Autodesk Inventor part; units mm, degrees
(part 2 of 3)
sketch "Эскиз30" plane through (0, 0, 0) normal (-1, 0, 0) x (0, 0, 1)
  circle A0 centre (-371.0468, 185.0848) radius 1.625 projected
  circle A1 centre (-103, 60) radius 2.1 projected
  circle A2 centre (-135.25, 60) radius 2.1 projected
  circle A3 centre (-173.9908, 56.343) radius 2.1 projected
  circle A4 centre (-50.8872, 165.0002) radius 2.1 projected
  circle A5 centre (-287, 56.343) radius 2.1 projected
  circle A6 centre (-319.1128, 165.0002) radius 2.1 projected
  arc A7 (-250, 372) -> (-253, 375) centre (-253, 372) ccw projected
  line L0 (-253, 375) -> (-377, 375) projected
  arc A8 (-377, 375) -> (-380, 372) centre (-377, 372) ccw projected
  line L1 (-380, 372) -> (-380, -2) projected
  arc A9 (-380, -2) -> (-377, -5) centre (-377, -2) ccw projected
  line L2 (-377, -5) -> (7, -5) projected
  arc A10 (7, -5) -> (10, -2) centre (7, -2) ccw projected
  line L3 (10, -2) -> (10, 372) projected
  arc A11 (10, 372) -> (7, 375) centre (7, 372) ccw projected
  line L4 (7, 375) -> (-117, 375) projected
  arc A12 (-117, 375) -> (-120, 372) centre (-117, 372) ccw projected
  line L5 (-120, 372) -> (-120, 323.5966) projected
  arc A13 (-123, 320.5966) -> (-120, 323.5966) centre (-123, 323.5966) ccw projected
  line L6 (-123, 320.5966) -> (-247, 320.5966) projected
  arc A14 (-250, 323.5966) -> (-247, 320.5966) centre (-247, 323.5966) ccw projected
  line L7 (-250, 323.5966) -> (-250, 372) projected
  arc A15 (-43, 338.848) -> (-40, 341.848) centre (-43, 341.848) ccw projected
  line L8 (-40, 341.848) -> (-40, 367) projected
  arc A16 (-37, 370) -> (-40, 367) centre (-37, 367) ccw projected
  line L9 (-37, 370) -> (-1, 370) projected
  arc A17 (2, 367) -> (-1, 370) centre (-1, 367) ccw projected
  line L10 (2, 367) -> (2, 269.848) projected
  arc A18 (-1, 266.848) -> (2, 269.848) centre (-1, 269.848) ccw projected
  line L11 (-1, 266.848) -> (-49, 266.848) projected
  arc A19 (-52, 269.848) -> (-49, 266.848) centre (-49, 269.848) ccw projected
  line L12 (-52, 269.848) -> (-52, 335.848) projected
  arc A20 (-49, 338.848) -> (-52, 335.848) centre (-49, 335.848) ccw projected
  line L13 (-49, 338.848) -> (-43, 338.848) projected
  arc A21 (-40, 28.152) -> (-43, 31.152) centre (-43, 28.152) ccw projected
  line L14 (-43, 31.152) -> (-49, 31.152) projected
  arc A22 (-52, 34.152) -> (-49, 31.152) centre (-49, 34.152) ccw projected
  line L15 (-52, 34.152) -> (-52, 100.152) projected
  arc A23 (-49, 103.152) -> (-52, 100.152) centre (-49, 100.152) ccw projected
  line L16 (-49, 103.152) -> (-43, 103.152) projected
  arc A24 (-43, 103.152) -> (-40, 106.152) centre (-43, 106.152) ccw projected
  line L17 (-40, 106.152) -> (-40, 160) projected
  arc A25 (-37, 163) -> (-40, 160) centre (-37, 160) ccw projected
  line L18 (-37, 163) -> (-1, 163) projected
  arc A26 (2, 160) -> (-1, 163) centre (-1, 160) ccw projected
  line L19 (2, 160) -> (2, 3) projected
  arc A27 (-1, 0) -> (2, 3) centre (-1, 3) ccw projected
  line L20 (-1, 0) -> (-37, 0) projected
  arc A28 (-40, 3) -> (-37, 0) centre (-37, 3) ccw projected
  line L21 (-40, 3) -> (-40, 28.152) projected
  line L22 (-165, 8) -> (-165, 44) projected
  arc A29 (-162, 47) -> (-165, 44) centre (-162, 44) ccw projected
  line L23 (-162, 47) -> (-96, 47) projected
  arc A30 (-93, 44) -> (-96, 47) centre (-96, 44) ccw projected
  line L24 (-93, 44) -> (-93, 8) projected
  arc A31 (-96, 5) -> (-93, 8) centre (-96, 8) ccw projected
  line L25 (-96, 5) -> (-162, 5) projected
  arc A32 (-165, 8) -> (-162, 5) centre (-162, 8) ccw projected
  circle A33 centre (-152.75, 251.9941) radius 2.1 projected
  circle A34 centre (-217.25, 118.0059) radius 2.1 projected
  circle A35 centre (-217.25, 57.0059) radius 2.1 projected
  circle A36 centre (-217.25, 251.9941) radius 2.1 projected
  circle A37 centre (-152.75, 312.9941) radius 2.1 projected
  circle A38 centre (-152.75, 118.0059) radius 2.1 projected
  circle A39 centre (-152.75, 57.0059) radius 2.1 projected
  circle A40 centre (-217.25, 312.9941) radius 2.1 projected
  circle A41 centre (-124.375, 193.0059) radius 2 projected
  circle A42 centre (-124.375, 129.0059) radius 2 projected
  line L26 (-98.825, 137.3849) -> (-98.825, 226.3849) projected
  arc A43 (-95.825, 229.3849) -> (-98.825, 226.3849) centre (-95.825, 226.3849) ccw projected
  line L27 (-95.825, 229.3849) -> (-87.825, 229.3849) projected
  arc A44 (-84.825, 226.3849) -> (-87.825, 229.3849) centre (-87.825, 226.3849) ccw projected
  line L28 (-84.825, 226.3849) -> (-84.825, 137.3849) projected
  arc A45 (-87.825, 134.3849) -> (-84.825, 137.3849) centre (-87.825, 137.3849) ccw projected
  line L29 (-87.825, 134.3849) -> (-95.825, 134.3849) projected
  arc A46 (-98.825, 137.3849) -> (-95.825, 134.3849) centre (-95.825, 137.3849) ccw projected
  line L30 (-358.5, 185.5001) -> (-358.5, 244.5001) projected
  arc A47 (-355.5, 247.5001) -> (-358.5, 244.5001) centre (-355.5, 244.5001) ccw projected
  line L31 (-355.5, 247.5001) -> (-335, 247.5001) projected
  arc A48 (-332, 244.5001) -> (-335, 247.5001) centre (-335, 244.5001) ccw projected
  line L32 (-332, 244.5001) -> (-332, 185.5001) projected
  arc A49 (-335, 182.5001) -> (-332, 185.5001) centre (-335, 185.5001) ccw projected
  line L33 (-335, 182.5001) -> (-355.5, 182.5001) projected
  arc A50 (-358.5, 185.5001) -> (-355.5, 182.5001) centre (-355.5, 185.5001) ccw projected
  line L34 (-35, 247.5001) -> (-14.5, 247.5001) projected
  arc A51 (-11.5, 244.5001) -> (-14.5, 247.5001) centre (-14.5, 244.5001) ccw projected
  line L35 (-11.5, 244.5001) -> (-11.5, 185.5001) projected
  arc A52 (-14.5, 182.5001) -> (-11.5, 185.5001) centre (-14.5, 185.5001) ccw projected
  line L36 (-14.5, 182.5001) -> (-35, 182.5001) projected
  arc A53 (-38, 185.5001) -> (-35, 182.5001) centre (-35, 185.5001) ccw projected
  line L37 (-38, 185.5001) -> (-38, 244.5001) projected
  arc A54 (-35, 247.5001) -> (-38, 244.5001) centre (-35, 244.5001) ccw projected
  arc A55 (-185, 192.7028) -> (-185, 193.309) centre (-183.175, 193.0059) ccw projected
  line L38 (-185, 192.7028) -> (-185, 193.309) projected
  circle A56 centre (-376, 368.9) radius 2.1 projected
  circle A57 centre (-299, 142) radius 1.625 projected
  circle A58 centre (-299, 2.0002) radius 1.625 projected
  circle A59 centre (-54, 368) radius 1.625 projected
  circle A60 centre (6, 1.1) radius 2.1 projected
  circle A61 centre (6, 368.9) radius 2.1 projected
  circle A62 centre (-54, 142) radius 1.625 projected
  circle A63 centre (1, 228) radius 1.625 projected
  circle A64 centre (-316, 2.0002) radius 1.625 projected
  circle A65 centre (-371, 228) radius 1.625 projected
  circle A66 centre (-299, 368) radius 1.625 projected
  circle A67 centre (-183.175, 129.0059) radius 1.85 projected
  circle A68 centre (-316, 228) radius 1.625 projected
  circle A69 centre (-316, 142) radius 1.625 projected
  circle A70 centre (-71, 228) radius 1.625 projected
  circle A71 centre (-71, 368) radius 1.625 projected
  circle A72 centre (-54, 2.0002) radius 1.625 projected
  circle A73 centre (-71, 2.0002) radius 1.625 projected
  circle A74 centre (-71, 142) radius 1.625 projected
  circle A75 centre (-54, 228) radius 1.625 projected
  circle A76 centre (-376, 1.1) radius 2.1 projected
  circle A77 centre (-299, 228) radius 1.625 projected
  circle A78 centre (-316, 368) radius 1.625 projected
  arc A79 (-330, 341.848) -> (-327, 338.848) centre (-327, 341.848) ccw projected
  line L39 (-327, 338.848) -> (-321, 338.848) projected
  arc A80 (-318, 335.848) -> (-321, 338.848) centre (-321, 335.848) ccw projected
  line L40 (-318, 335.848) -> (-318, 269.848) projected
  arc A81 (-321, 266.848) -> (-318, 269.848) centre (-321, 269.848) ccw projected
  line L41 (-321, 266.848) -> (-369, 266.848) projected
  arc A82 (-372, 269.848) -> (-369, 266.848) centre (-369, 269.848) ccw projected
  line L42 (-372, 269.848) -> (-372, 367) projected
  arc A83 (-369, 370) -> (-372, 367) centre (-369, 367) ccw projected
  line L43 (-369, 370) -> (-333, 370) projected
  arc A84 (-330, 367) -> (-333, 370) centre (-333, 367) ccw projected
  line L44 (-330, 367) -> (-330, 341.848) projected
  arc A85 (-327, 31.152) -> (-330, 28.152) centre (-327, 28.152) ccw projected
  line L45 (-330, 28.152) -> (-330, 3) projected
  arc A86 (-333, 0) -> (-330, 3) centre (-333, 3) ccw projected
  line L46 (-333, 0) -> (-369, 0) projected
  arc A87 (-372, 3) -> (-369, 0) centre (-369, 3) ccw projected
  line L47 (-372, 3) -> (-372, 160) projected
  arc A88 (-369, 163) -> (-372, 160) centre (-369, 160) ccw projected
  line L48 (-369, 163) -> (-333, 163) projected
  arc A89 (-330, 160) -> (-333, 163) centre (-333, 160) ccw projected
  line L49 (-330, 160) -> (-330, 106.152) projected
  arc A90 (-330, 106.152) -> (-327, 103.152) centre (-327, 106.152) ccw projected
  line L50 (-327, 103.152) -> (-321, 103.152) projected
  arc A91 (-318, 100.152) -> (-321, 103.152) centre (-321, 100.152) ccw projected
  line L51 (-318, 100.152) -> (-318, 34.152) projected
  arc A92 (-321, 31.152) -> (-318, 34.152) centre (-321, 34.152) ccw projected
  line L52 (-321, 31.152) -> (-327, 31.152) projected
  line L53 (-224.75, 65.0059) -> (-224.75, 110.0059) projected
  line L54 (-282, 51.343) -> (-282, 61.343) projected
  line L55 (-268.3252, 69.343) -> (-228.25, 69.343)
  line L56 (-226.25, 71.343) -> (-226.25, 99.9959)
  line L57 (-235.9248, 106.343) -> (-276, 106.343)
  line L58 (-278, 104.343) -> (-278, 75.6902)
  line L59 (-278, 69.343) -> (-226.25, 106.343)
  line L60 (-269.4885, 72.97) -> (-229.4132, 101.6228)
  line L61 (-274.8368, 74.0633) -> (-234.7615, 102.7161)
  arc A93 (-269.4885, 72.97) -> (-268.3252, 69.343) centre (-268.3252, 71.343) ccw
  arc A94 (-278, 75.6902) -> (-274.8368, 74.0633) centre (-276, 75.6902) ccw
  arc A95 (-234.7615, 102.7161) -> (-235.9248, 106.343) centre (-235.9248, 104.343) ccw
  arc A96 (-276, 106.343) -> (-278, 104.343) centre (-276, 104.343) ccw
  arc A97 (-228.25, 69.343) -> (-226.25, 71.343) centre (-228.25, 71.343) ccw
  arc A98 (-226.25, 99.9959) -> (-229.4132, 101.6228) centre (-228.25, 99.9959) ccw
  line L62 (-185, -235.3635) -> (-185, 601.2713)
  line L63 (-101.6748, 69.343) -> (-141.75, 69.343)
  line L64 (-143.75, 71.343) -> (-143.75, 99.9959)
  line L65 (-134.0752, 106.343) -> (-94, 106.343)
  line L66 (-92, 104.343) -> (-92, 75.6902)
  line L67 (-92, 69.343) -> (-143.75, 106.343)
  line L68 (-100.5115, 72.97) -> (-140.5868, 101.6228)
  line L69 (-95.1632, 74.0633) -> (-135.2385, 102.7161)
  arc A99 (-101.6748, 69.343) -> (-100.5115, 72.97) centre (-101.6748, 71.343) ccw
  arc A100 (-95.1632, 74.0633) -> (-92, 75.6902) centre (-94, 75.6902) ccw
  arc A101 (-134.0752, 106.343) -> (-135.2385, 102.7161) centre (-134.0752, 104.343) ccw
  arc A102 (-92, 104.343) -> (-94, 106.343) centre (-94, 104.343) ccw
  arc A103 (-143.75, 71.343) -> (-141.75, 69.343) centre (-141.75, 71.343) ccw
  arc A104 (-140.5868, 101.6228) -> (-143.75, 99.9959) centre (-141.75, 99.9959) ccw
  line L70 (-268.3252, 133.343) -> (-228.25, 133.343)
  line L71 (-226.25, 135.343) -> (-226.25, 163.9959)
  line L72 (-235.9248, 170.343) -> (-276, 170.343)
  line L73 (-278, 168.343) -> (-278, 139.6902)
  line L74 (-278, 133.343) -> (-226.25, 170.343)
  line L75 (-269.4885, 136.97) -> (-229.4132, 165.6228)
  line L76 (-274.8368, 138.0633) -> (-234.7615, 166.7161)
  arc A105 (-269.4885, 136.97) -> (-268.3252, 133.343) centre (-268.3252, 135.343) ccw
  arc A106 (-278, 139.6902) -> (-274.8368, 138.0633) centre (-276, 139.6902) ccw
  arc A107 (-234.7615, 166.7161) -> (-235.9248, 170.343) centre (-235.9248, 168.343) ccw
  arc A108 (-276, 170.343) -> (-278, 168.343) centre (-276, 168.343) ccw
  arc A109 (-228.25, 133.343) -> (-226.25, 135.343) centre (-228.25, 135.343) ccw
  arc A110 (-226.25, 163.9959) -> (-229.4132, 165.6228) centre (-228.25, 163.9959) ccw
  line L77 (-458.8698, 185) -> (88.8698, 185) projected
  line L78 (-268.3252, 300.657) -> (-228.25, 300.657)
  line L79 (-226.25, 298.657) -> (-226.25, 270.0041)
  line L80 (-235.9248, 263.657) -> (-276, 263.657)
  line L81 (-278, 265.657) -> (-278, 294.3098)
  line L82 (-278, 300.657) -> (-226.25, 263.657)
  line L83 (-269.4885, 297.03) -> (-229.4132, 268.3772)
  line L84 (-274.8368, 295.9367) -> (-234.7615, 267.2839)
  arc A111 (-268.3252, 300.657) -> (-269.4885, 297.03) centre (-268.3252, 298.657) ccw
  arc A112 (-274.8368, 295.9367) -> (-278, 294.3098) centre (-276, 294.3098) ccw
  arc A113 (-235.9248, 263.657) -> (-234.7615, 267.2839) centre (-235.9248, 265.657) ccw
  arc A114 (-278, 265.657) -> (-276, 263.657) centre (-276, 265.657) ccw
  arc A115 (-226.25, 298.657) -> (-228.25, 300.657) centre (-228.25, 298.657) ccw
  arc A116 (-229.4132, 268.3772) -> (-226.25, 270.0041) centre (-228.25, 270.0041) ccw
  line L85 (-134.0752, 263.657) -> (-94, 263.657)
  arc A117 (-94, 263.657) -> (-92, 265.657) centre (-94, 265.657) ccw
  arc A118 (-135.2385, 267.2839) -> (-134.0752, 263.657) centre (-134.0752, 265.657) ccw
  arc A119 (-143.75, 270.0041) -> (-140.5868, 268.3772) centre (-141.75, 270.0041) ccw
  line L86 (-92, 265.657) -> (-92, 294.3098)
  line L87 (-95.1632, 295.9367) -> (-135.2385, 267.2839)
  line L88 (-92, 300.657) -> (-143.75, 263.657)
  arc A120 (-100.5115, 297.03) -> (-101.6748, 300.657) centre (-101.6748, 298.657) ccw
  arc A121 (-92, 294.3098) -> (-95.1632, 295.9367) centre (-94, 294.3098) ccw
  line L89 (-101.6748, 300.657) -> (-141.75, 300.657)
  line L90 (-143.75, 298.657) -> (-143.75, 270.0041)
  arc A122 (-141.75, 300.657) -> (-143.75, 298.657) centre (-141.75, 298.657) ccw
  line L91 (-100.5115, 297.03) -> (-140.5868, 268.3772)
  arc A123 (-226.25, 230.3098) -> (-229.4132, 231.9367) centre (-228.25, 230.3098) ccw
  line L92 (-226.25, 201.657) -> (-226.25, 230.3098)
  arc A124 (-228.25, 199.657) -> (-226.25, 201.657) centre (-228.25, 201.657) ccw
  arc A125 (-278, 206.0041) -> (-274.8368, 204.3772) centre (-276, 206.0041) ccw
  arc A126 (-269.4885, 203.2839) -> (-268.3252, 199.657) centre (-268.3252, 201.657) ccw
  line L93 (-278, 234.657) -> (-278, 206.0041)
  arc A127 (-276, 236.657) -> (-278, 234.657) centre (-276, 234.657) ccw
  line L94 (-268.3252, 199.657) -> (-228.25, 199.657)
  line L95 (-235.9248, 236.657) -> (-276, 236.657)
  arc A128 (-234.7615, 233.03) -> (-235.9248, 236.657) centre (-235.9248, 234.657) ccw
  line L96 (-269.4885, 203.2839) -> (-229.4132, 231.9367)
  line L97 (-278, 199.657) -> (-226.25, 236.657)
  line L98 (-274.8368, 204.3772) -> (-234.7615, 233.03)
  arc A129 (-130.725, 234.2716) -> (-133.9769, 235.8314) centre (-132.725, 234.2716) ccw
  line L99 (-130.725, 206.0059) -> (-130.725, 234.2716)
  arc A130 (-138.3555, 237.4461) -> (-139.6074, 241.0059) centre (-139.6074, 239.0059) ccw
  line L100 (-167.9426, 204.0059) -> (-132.725, 204.0059)
  arc A131 (-169.1945, 207.5656) -> (-167.9426, 204.0059) centre (-167.9426, 206.0059) ccw
  line L101 (-169.1945, 207.5656) -> (-133.9769, 235.8314)
  line L102 (-176.825, 204.0059) -> (-130.725, 241.0059)
  line L103 (-173.5731, 209.1803) -> (-138.3555, 237.4461)
  line L104 (-139.6074, 241.0059) -> (-174.825, 241.0059)
  arc A132 (-176.825, 210.7401) -> (-173.5731, 209.1803) centre (-174.825, 210.7401) ccw
  line L105 (-176.825, 239.0059) -> (-176.825, 210.7401)
  arc A133 (-174.825, 241.0059) -> (-176.825, 239.0059) centre (-174.825, 239.0059) ccw
  arc A134 (-132.725, 204.0059) -> (-130.725, 206.0059) centre (-132.725, 206.0059) ccw
  line L106 (-130.725, 182.9338) -> (-130.725, 189.1279) projected
  point P0 (0, 0)
  point P1 (-145.25, 110.0059)
  point P2 (-255.9624, 106.343)
  point P3 (-224.75, 259.9941)
  point P4 (-145.25, 259.9941)
  point P5 (-255.9624, 263.657)
  point P6 (-226.25, 149.6695)
  point P7 (-176.825, 195.5059)
  dimension "d123" = 9
  dimension "d124" = 9
  dimension "d125" = 37
  dimension "d126" = 2
  dimension "d127" = 2
  dimension "d128" = 2
  dimension "d129" = 37
  dimension "d130" = 2
  dimension "d131" = 2
  dimension "d132" = 2
  dimension "d133" = 0
  dimension "d141" = 27
  dimension "d142" = 37
  dimension "d143" = 2
  dimension "d144" = 2
  dimension "d145" = 2
  dimension "d146" = 27
  dimension "d147" = 0
  dimension "d148" = 0
  dimension "d149" = 37
  dimension "d150" = 2
  dimension "d151" = 2
  dimension "d152" = 2
  dimension "d153" = 11
  dimension "d154" = 0
  dimension "d155" = 0
  constraints: 100 end point, 84 point on circle, 64 symmetric about line, 48 tangent, 42 centre point, 28 point on line, 20 equal radius, 16 parallel, 5 horizontal, 4 perpendicular, 2 midpoint, 1 vertical, 21 other
  measures "d123" distance from line of L58 A5.centre
  measures "d124" distance from line of A35.centre L56
  measures "d125" distance between parallel lines of L57 L55
  measures "d126" distance between parallel lines of L59 L60
  measures "d127" distance between parallel lines of L59 L61
  measures "d128" radius of A93
  measures "d129" distance between parallel lines of L72 L70
  measures "d130" distance between parallel lines of L74 L75
  measures "d131" distance between parallel lines of L74 L76
  measures "d132" radius of A105
  measures "d133" distance between parallel lines of L58 L73
  measures "d141" distance between parallel lines of L57 L70
  measures "d142" distance between parallel lines of L95 L94
  measures "d143" distance between parallel lines of L97 L96
  measures "d144" distance between parallel lines of L97 L98
  measures "d145" radius of A126
  measures "d146" distance between parallel lines of L95 L80
  measures "d147" distance between parallel lines of L73 L93
  measures "d148" distance from line of point (-226.25, 149.669) L92
  measures "d149" distance between parallel lines of L104 L100
  measures "d150" distance between parallel lines of L102 L101
  measures "d151" distance between parallel lines of L102 L103
  measures "d152" radius of A131
  measures "d153" distance from line of A55.centre L100
  measures "d154" distance from line of point (-176.825, 195.506) L105
  measures "d155" distance between parallel lines of L106 L99
extrude "Выдавливание27" cut sketch "Эскиз30" against normal blind 10 contours A93 L60 A98 L56 A97 L55 | A95 L61 A94 L58 A96 L57 | L63 A103 L64 A104 L68 A99 | L65 A102 L66 A100 L69 A101 | A105 L75 A110 L71 A109 L70 | A107 L76 A106 L73 A108 L72 | L78 A115 L79 A116 L83 A111 | L80 A114 L81 A112 L84 A113 | A118 L87 A121 L86 A117 L85 | L90 A122 L89 A120 L91 A119 | L92 A124 L94 A126 L96 A123 | L93 A127 L95 A128 L98 A125 | L99 A134 L100 A131 L101 A129 | L103 A132 L105 A133 L104 A130
sketch "Эскиз31" plane through (1.5, 0, 0) normal (1, 0, 0) x (0, 0, -1)
  point P0 (0, 0)
sketch "Эскиз32" plane through (1.5, 0, 0) normal (1, 0, 0) x (0, 0, -1)
  arc A0 (278, 234.657) -> (276, 236.657) centre (276, 234.657) ccw projected
  line L0 (278, 234.657) -> (278, 206.0041) projected
  arc A1 (274.8368, 204.3772) -> (278, 206.0041) centre (276, 206.0041) ccw projected
  line L1 (274.8368, 204.3772) -> (234.7615, 233.03) projected
  arc A2 (235.9248, 236.657) -> (234.7615, 233.03) centre (235.9248, 234.657) ccw projected
  line L2 (235.9248, 236.657) -> (276, 236.657) projected
  line L3 (278, 104.343) -> (278, 75.6902) projected
  arc A3 (274.8368, 74.0633) -> (278, 75.6902) centre (276, 75.6902) ccw projected
  line L4 (274.8368, 74.0633) -> (234.7615, 102.7161) projected
  arc A4 (235.9248, 106.343) -> (234.7615, 102.7161) centre (235.9248, 104.343) ccw projected
  line L5 (235.9248, 106.343) -> (276, 106.343) projected
  arc A5 (278, 104.343) -> (276, 106.343) centre (276, 104.343) ccw projected
  line L6 (176.825, 239.0059) -> (176.825, 210.7401) projected
  arc A6 (173.5731, 209.1803) -> (176.825, 210.7401) centre (174.825, 210.7401) ccw projected
  line L7 (173.5731, 209.1803) -> (138.3555, 237.4461) projected
  arc A7 (139.6074, 241.0059) -> (138.3555, 237.4461) centre (139.6074, 239.0059) ccw projected
  line L8 (139.6074, 241.0059) -> (174.825, 241.0059) projected
  arc A8 (176.825, 239.0059) -> (174.825, 241.0059) centre (174.825, 239.0059) ccw projected
  arc A9 (143.75, 298.657) -> (141.75, 300.657) centre (141.75, 298.657) ccw projected
  line L9 (143.75, 298.657) -> (143.75, 270.0041) projected
  arc A10 (140.5868, 268.3772) -> (143.75, 270.0041) centre (141.75, 270.0041) ccw projected
  line L10 (140.5868, 268.3772) -> (100.5115, 297.03) projected
  arc A11 (101.6748, 300.657) -> (100.5115, 297.03) centre (101.6748, 298.657) ccw projected
  line L11 (101.6748, 300.657) -> (141.75, 300.657) projected
  arc A12 (143.75, 99.9959) -> (140.5868, 101.6228) centre (141.75, 99.9959) ccw projected
  line L12 (143.75, 99.9959) -> (143.75, 71.343) projected
  arc A13 (141.75, 69.343) -> (143.75, 71.343) centre (141.75, 71.343) ccw projected
  line L13 (141.75, 69.343) -> (101.6748, 69.343) projected
  arc A14 (100.5115, 72.97) -> (101.6748, 69.343) centre (101.6748, 71.343) ccw projected
  line L14 (100.5115, 72.97) -> (140.5868, 101.6228) projected
  arc A15 (226.25, 135.343) -> (228.25, 133.343) centre (228.25, 135.343) ccw projected
  line L15 (226.25, 135.343) -> (226.25, 163.9959) projected
  arc A16 (229.4132, 165.6228) -> (226.25, 163.9959) centre (228.25, 163.9959) ccw projected
  line L16 (229.4132, 165.6228) -> (269.4885, 136.97) projected
  arc A17 (268.3252, 133.343) -> (269.4885, 136.97) centre (268.3252, 135.343) ccw projected
  line L17 (268.3252, 133.343) -> (228.25, 133.343) projected
  arc A18 (278, 294.3098) -> (274.8368, 295.9367) centre (276, 294.3098) ccw projected
  line L18 (278, 294.3098) -> (278, 265.657) projected
  arc A19 (276, 263.657) -> (278, 265.657) centre (276, 265.657) ccw projected
  line L19 (276, 263.657) -> (235.9248, 263.657) projected
  arc A20 (234.7615, 267.2839) -> (235.9248, 263.657) centre (235.9248, 265.657) ccw projected
  line L20 (234.7615, 267.2839) -> (274.8368, 295.9367) projected
  arc A21 (226.25, 201.657) -> (228.25, 199.657) centre (228.25, 201.657) ccw projected
  line L21 (226.25, 201.657) -> (226.25, 230.3098) projected
  arc A22 (229.4132, 231.9367) -> (226.25, 230.3098) centre (228.25, 230.3098) ccw projected
  line L22 (229.4132, 231.9367) -> (269.4885, 203.2839) projected
  arc A23 (268.3252, 199.657) -> (269.4885, 203.2839) centre (268.3252, 201.657) ccw projected
  line L23 (268.3252, 199.657) -> (228.25, 199.657) projected
  arc A24 (226.25, 71.343) -> (228.25, 69.343) centre (228.25, 71.343) ccw projected
  line L24 (226.25, 71.343) -> (226.25, 99.9959) projected
  arc A25 (229.4132, 101.6228) -> (226.25, 99.9959) centre (228.25, 99.9959) ccw projected
  line L25 (229.4132, 101.6228) -> (269.4885, 72.97) projected
  arc A26 (268.3252, 69.343) -> (269.4885, 72.97) centre (268.3252, 71.343) ccw projected
  line L26 (268.3252, 69.343) -> (228.25, 69.343) projected
  arc A27 (130.725, 206.0059) -> (132.725, 204.0059) centre (132.725, 206.0059) ccw projected
  line L27 (130.725, 206.0059) -> (130.725, 234.2716) projected
  arc A28 (133.9769, 235.8314) -> (130.725, 234.2716) centre (132.725, 234.2716) ccw projected
  line L28 (133.9769, 235.8314) -> (169.1945, 207.5656) projected
  arc A29 (167.9426, 204.0059) -> (169.1945, 207.5656) centre (167.9426, 206.0059) ccw projected
  line L29 (167.9426, 204.0059) -> (132.725, 204.0059) projected
  arc A30 (92, 265.657) -> (94, 263.657) centre (94, 265.657) ccw projected
  line L30 (92, 265.657) -> (92, 294.3098) projected
  arc A31 (95.1632, 295.9367) -> (92, 294.3098) centre (94, 294.3098) ccw projected
  line L31 (95.1632, 295.9367) -> (135.2385, 267.2839) projected
  arc A32 (134.0752, 263.657) -> (135.2385, 267.2839) centre (134.0752, 265.657) ccw projected
  line L32 (134.0752, 263.657) -> (94, 263.657) projected
  arc A33 (94, 106.343) -> (92, 104.343) centre (94, 104.343) ccw projected
  line L33 (94, 106.343) -> (134.0752, 106.343) projected
  arc A34 (135.2385, 102.7161) -> (134.0752, 106.343) centre (134.0752, 104.343) ccw projected
  line L34 (135.2385, 102.7161) -> (95.1632, 74.0633) projected
  arc A35 (92, 75.6902) -> (95.1632, 74.0633) centre (94, 75.6902) ccw projected
  line L35 (92, 75.6902) -> (92, 104.343) projected
  arc A36 (235.9248, 170.343) -> (234.7615, 166.7161) centre (235.9248, 168.343) ccw projected
  line L36 (235.9248, 170.343) -> (276, 170.343) projected
  arc A37 (278, 168.343) -> (276, 170.343) centre (276, 168.343) ccw projected
  line L37 (278, 168.343) -> (278, 139.6902) projected
  arc A38 (274.8368, 138.0633) -> (278, 139.6902) centre (276, 139.6902) ccw projected
  line L38 (274.8368, 138.0633) -> (234.7615, 166.7161) projected
  line L39 (226.25, 270.0041) -> (226.25, 298.657) projected
  arc A39 (228.25, 300.657) -> (226.25, 298.657) centre (228.25, 298.657) ccw projected
  line L40 (228.25, 300.657) -> (268.3252, 300.657) projected
  arc A40 (269.4885, 297.03) -> (268.3252, 300.657) centre (268.3252, 298.657) ccw projected
  line L41 (269.4885, 297.03) -> (229.4132, 268.3772) projected
  arc A41 (226.25, 270.0041) -> (229.4132, 268.3772) centre (228.25, 270.0041) ccw projected
  circle A42 centre (371.0468, 185.0848) radius 1.625 projected
  circle A43 centre (103, 60) radius 2.1 projected
  circle A44 centre (135.25, 60) radius 2.1 projected
  circle A45 centre (173.9908, 56.343) radius 2.1 projected
  circle A46 centre (50.8872, 165.0002) radius 2.1 projected
  circle A47 centre (287, 56.343) radius 2.1 projected
  circle A48 centre (319.1128, 165.0002) radius 2.1 projected
  arc A49 (40, 341.848) -> (43, 338.848) centre (43, 341.848) ccw projected
  line L42 (43, 338.848) -> (49, 338.848) projected
  arc A50 (52, 335.848) -> (49, 338.848) centre (49, 335.848) ccw projected
  line L43 (52, 335.848) -> (52, 269.848) projected
  arc A51 (49, 266.848) -> (52, 269.848) centre (49, 269.848) ccw projected
  line L44 (49, 266.848) -> (1, 266.848) projected
  arc A52 (-2, 269.848) -> (1, 266.848) centre (1, 269.848) ccw projected
  line L45 (-2, 269.848) -> (-2, 367) projected
  arc A53 (1, 370) -> (-2, 367) centre (1, 367) ccw projected
  line L46 (1, 370) -> (37, 370) projected
  arc A54 (40, 367) -> (37, 370) centre (37, 367) ccw projected
  line L47 (40, 367) -> (40, 341.848) projected
  arc A55 (253, 375) -> (250, 372) centre (253, 372) ccw projected
  line L48 (250, 372) -> (250, 323.5966) projected
  arc A56 (247, 320.5966) -> (250, 323.5966) centre (247, 323.5966) ccw projected
  line L49 (247, 320.5966) -> (123, 320.5966) projected
  arc A57 (120, 323.5966) -> (123, 320.5966) centre (123, 323.5966) ccw projected
  line L50 (120, 323.5966) -> (120, 372) projected
  arc A58 (120, 372) -> (117, 375) centre (117, 372) ccw projected
  line L51 (117, 375) -> (-7, 375) projected
  arc A59 (-7, 375) -> (-10, 372) centre (-7, 372) ccw projected
  line L52 (-10, 372) -> (-10, -2) projected
  arc A60 (-10, -2) -> (-7, -5) centre (-7, -2) ccw projected
  line L53 (-7, -5) -> (377, -5) projected
  arc A61 (377, -5) -> (380, -2) centre (377, -2) ccw projected
  line L54 (380, -2) -> (380, 372) projected
  arc A62 (380, 372) -> (377, 375) centre (377, 372) ccw projected
  line L55 (377, 375) -> (253, 375) projected
  arc A63 (327, 338.848) -> (330, 341.848) centre (327, 341.848) ccw projected
  line L56 (330, 341.848) -> (330, 367) projected
  arc A64 (333, 370) -> (330, 367) centre (333, 367) ccw projected
  line L57 (333, 370) -> (369, 370) projected
  arc A65 (372, 367) -> (369, 370) centre (369, 367) ccw projected
  line L58 (372, 367) -> (372, 269.848) projected
  arc A66 (369, 266.848) -> (372, 269.848) centre (369, 269.848) ccw projected
  line L59 (369, 266.848) -> (321, 266.848) projected
  arc A67 (318, 269.848) -> (321, 266.848) centre (321, 269.848) ccw projected
  line L60 (318, 269.848) -> (318, 335.848) projected
  arc A68 (321, 338.848) -> (318, 335.848) centre (321, 335.848) ccw projected
  line L61 (321, 338.848) -> (327, 338.848) projected
  line L62 (165, 44) -> (165, 8) projected
  arc A69 (162, 5) -> (165, 8) centre (162, 8) ccw projected
  line L63 (162, 5) -> (96, 5) projected
  arc A70 (93, 8) -> (96, 5) centre (96, 8) ccw projected
  line L64 (93, 8) -> (93, 44) projected
  arc A71 (96, 47) -> (93, 44) centre (96, 44) ccw projected
  line L65 (96, 47) -> (162, 47) projected
  arc A72 (165, 44) -> (162, 47) centre (162, 44) ccw projected
  circle A73 centre (152.75, 251.9941) radius 2.1 projected
  circle A74 centre (217.25, 118.0059) radius 2.1 projected
  circle A75 centre (217.25, 57.0059) radius 2.1 projected
  circle A76 centre (217.25, 251.9941) radius 2.1 projected
  circle A77 centre (152.75, 312.9941) radius 2.1 projected
  circle A78 centre (152.75, 118.0059) radius 2.1 projected
  circle A79 centre (152.75, 57.0059) radius 2.1 projected
  circle A80 centre (217.25, 312.9941) radius 2.1 projected
  circle A81 centre (124.375, 193.0059) radius 2 projected
  circle A82 centre (124.375, 129.0059) radius 2 projected
  line L66 (98.825, 226.3849) -> (98.825, 137.3849) projected
  arc A83 (95.825, 134.3849) -> (98.825, 137.3849) centre (95.825, 137.3849) ccw projected
  line L67 (95.825, 134.3849) -> (87.825, 134.3849) projected
  arc A84 (84.825, 137.3849) -> (87.825, 134.3849) centre (87.825, 137.3849) ccw projected
  line L68 (84.825, 137.3849) -> (84.825, 226.3849) projected
  arc A85 (87.825, 229.3849) -> (84.825, 226.3849) centre (87.825, 226.3849) ccw projected
  line L69 (87.825, 229.3849) -> (95.825, 229.3849) projected
  arc A86 (98.825, 226.3849) -> (95.825, 229.3849) centre (95.825, 226.3849) ccw projected
  line L70 (358.5, 244.5001) -> (358.5, 185.5001) projected
  arc A87 (355.5, 182.5001) -> (358.5, 185.5001) centre (355.5, 185.5001) ccw projected
  line L71 (355.5, 182.5001) -> (335, 182.5001) projected
  arc A88 (332, 185.5001) -> (335, 182.5001) centre (335, 185.5001) ccw projected
  line L72 (332, 185.5001) -> (332, 244.5001) projected
  arc A89 (335, 247.5001) -> (332, 244.5001) centre (335, 244.5001) ccw projected
  line L73 (335, 247.5001) -> (355.5, 247.5001) projected
  arc A90 (358.5, 244.5001) -> (355.5, 247.5001) centre (355.5, 244.5001) ccw projected
  line L74 (14.5, 247.5001) -> (35, 247.5001) projected
  arc A91 (38, 244.5001) -> (35, 247.5001) centre (35, 244.5001) ccw projected
  line L75 (38, 244.5001) -> (38, 185.5001) projected
  arc A92 (35, 182.5001) -> (38, 185.5001) centre (35, 185.5001) ccw projected
  line L76 (35, 182.5001) -> (14.5, 182.5001) projected
  arc A93 (11.5, 185.5001) -> (14.5, 182.5001) centre (14.5, 185.5001) ccw projected
  line L77 (11.5, 185.5001) -> (11.5, 244.5001) projected
  arc A94 (14.5, 247.5001) -> (11.5, 244.5001) centre (14.5, 244.5001) ccw projected
  arc A95 (185, 193.309) -> (185, 192.7028) centre (183.175, 193.0059) ccw projected
  line L78 (185, 193.309) -> (185, 192.7028) projected
  circle A96 centre (376, 368.9) radius 2.1 projected
  circle A97 centre (299, 142) radius 1.625 projected
  circle A98 centre (299, 2.0002) radius 1.625 projected
  circle A99 centre (54, 368) radius 1.625 projected
  circle A100 centre (-6, 1.1) radius 2.1 projected
  circle A101 centre (-6, 368.9) radius 2.1 projected
  circle A102 centre (54, 142) radius 1.625 projected
  circle A103 centre (-1, 228) radius 1.625 projected
  circle A104 centre (316, 2.0002) radius 1.625 projected
  circle A105 centre (371, 228) radius 1.625 projected
  circle A106 centre (299, 368) radius 1.625 projected
  circle A107 centre (183.175, 129.0059) radius 1.85 projected
  circle A108 centre (316, 228) radius 1.625 projected
  circle A109 centre (316, 142) radius 1.625 projected
  circle A110 centre (71, 228) radius 1.625 projected
  circle A111 centre (71, 368) radius 1.625 projected
  circle A112 centre (54, 2.0002) radius 1.625 projected
  circle A113 centre (71, 2.0002) radius 1.625 projected
  circle A114 centre (71, 142) radius 1.625 projected
  circle A115 centre (54, 228) radius 1.625 projected
  circle A116 centre (376, 1.1) radius 2.1 projected
  circle A117 centre (299, 228) radius 1.625 projected
  circle A118 centre (316, 368) radius 1.625 projected
  arc A119 (43, 31.152) -> (40, 28.152) centre (43, 28.152) ccw projected
  line L79 (40, 28.152) -> (40, 3) projected
  arc A120 (37, 0) -> (40, 3) centre (37, 3) ccw projected
  line L80 (37, 0) -> (1, 0) projected
  arc A121 (-2, 3) -> (1, 0) centre (1, 3) ccw projected
  line L81 (-2, 3) -> (-2, 160) projected
  arc A122 (1, 163) -> (-2, 160) centre (1, 160) ccw projected
  line L82 (1, 163) -> (37, 163) projected
  arc A123 (40, 160) -> (37, 163) centre (37, 160) ccw projected
  line L83 (40, 160) -> (40, 106.152) projected
  arc A124 (40, 106.152) -> (43, 103.152) centre (43, 106.152) ccw projected
  line L84 (43, 103.152) -> (49, 103.152) projected
  arc A125 (52, 100.152) -> (49, 103.152) centre (49, 100.152) ccw projected
  line L85 (52, 100.152) -> (52, 34.152) projected
  arc A126 (49, 31.152) -> (52, 34.152) centre (49, 34.152) ccw projected
  line L86 (49, 31.152) -> (43, 31.152) projected
  arc A127 (330, 28.152) -> (327, 31.152) centre (327, 28.152) ccw projected
  line L87 (327, 31.152) -> (321, 31.152) projected
  arc A128 (318, 34.152) -> (321, 31.152) centre (321, 34.152) ccw projected
  line L88 (318, 34.152) -> (318, 100.152) projected
  arc A129 (321, 103.152) -> (318, 100.152) centre (321, 100.152) ccw projected
  line L89 (321, 103.152) -> (327, 103.152) projected
  arc A130 (327, 103.152) -> (330, 106.152) centre (327, 106.152) ccw projected
  line L90 (330, 106.152) -> (330, 160) projected
  arc A131 (333, 163) -> (330, 160) centre (333, 160) ccw projected
  line L91 (333, 163) -> (369, 163) projected
  arc A132 (372, 160) -> (369, 163) centre (369, 160) ccw projected
  line L92 (372, 160) -> (372, 3) projected
  arc A133 (369, 0) -> (372, 3) centre (369, 3) ccw projected
  line L93 (369, 0) -> (333, 0) projected
  arc A134 (330, 3) -> (333, 0) centre (333, 3) ccw projected
  line L94 (330, 3) -> (330, 28.152) projected
  line L95 (120, 375) -> (78, 375)
  line L96 (78, 375) -> (78, 320.5966)
  line L97 (78, 320.5966) -> (120, 320.5966)
  line L98 (120, 320.5966) -> (120, 375)
  line L99 (78, 375) -> (292, 375)
  line L100 (292, 375) -> (292, 320.5966)
  line L101 (292, 320.5966) -> (78, 320.5966)
  line L102 (78, 320.5966) -> (78, 375)
  point P0 (0, 0)
  dimension "d158" = 42
  dimension "d159" = 42
  constraints: 16 end point, 4 parallel, 2 horizontal, 2 perpendicular, 1 point on line
  measures "d158" distance of L97.end L96.end
  measures "d159" distance between parallel lines of L48 L100
extrude "Выдавливание28" cut sketch "Эскиз32" against normal blind 10 contours L55 L100 L101 A56 L48 A55 | A55 L48 A56 L49 A57 L50 L98 L99 | L98 A58 L95 | A58 L50 L98 L97 L96 L51 | A57 L101 L98
fillet "Сопряжение2" radius 3 4 edges at (0.75, 375, -78) (0.75, 320.5966, -78) (0.75, 375, -292) (0.75, 320.5966, -292)
sketch "Эскиз33" plane through (1.5, 0, 0) normal (1, 0, 0) x (0, 0, -1)
  line L0 (-7, -5) -> (377, -5) projected
  line L1 (377, 375) -> (295, 375) projected
  line L2 (-18, 372) -> (-18, -2)
  line L3 (-10, -2) -> (-10, 372)
  line L4 (-15, 375) -> (-7, 375)
  arc A0 (-7, 375) -> (-10, 372) centre (-7, 372) ccw projected
  arc A1 (-7, 375) -> (-10, 372) centre (-7, 372) ccw
  line L5 (-15, -5) -> (-7, -5)
  arc A2 (-10, -2) -> (-7, -5) centre (-7, -2) ccw
  line L6 (388, 372) -> (388, -2)
  line L7 (380, -2) -> (380, 372)
  line L8 (385, -5) -> (377, -5)
  arc A3 (377, -5) -> (380, -2) centre (377, -2) ccw
  line L9 (377, 375) -> (385, 375)
  arc A4 (380, 372) -> (377, 375) centre (377, 372) ccw projected
  arc A5 (380, 372) -> (377, 375) centre (377, 372) ccw
  arc A6 (-15, 375) -> (-18, 372) centre (-15, 372) ccw
  arc A7 (-18, -2) -> (-15, -5) centre (-15, -2) ccw
  arc A8 (385, -5) -> (388, -2) centre (385, -2) ccw
  arc A9 (388, 372) -> (385, 375) centre (385, 372) ccw
  point P0 (0, 0)
  point P1 (-18, -5)
  point P2 (-18, 375)
  point P3 (388, 375)
  point P4 (388, -5)
  dimension "d163" = 380
  dimension "d202" = 3
  constraints: 19 point on circle, 16 end point, 8 centre point, 8 point on line, 8 tangent, 4 equal radius, 2 horizontal, 2 parallel
  measures "d163" distance between parallel lines of L0 L1
  measures "d202" radius of A6
extrude "Выдавливание29" add sketch "Эскиз33" against normal blind 1.5
sketch "Эскиз34" plane through (1.5, 0, 0) normal (1, 0, 0) x (0, 0, -1)
  line L0 (-18, -2) -> (-18, 372) projected
  line L1 (295, 375) -> (75, 375) projected
  line L2 (185, 375) -> (185, -494)
  circle A0 centre (371.0468, 185.0848) radius 1.625
  circle A1 centre (371.0468, 185.0848) radius 1.625 projected
  circle A2 centre (-1.0468, 185.0848) radius 1.625
  point P0 (0, 0)
  point P1 (-18, -5)
  point P2 (-18, 375)
  dimension "d172" = 3.25
  constraints: 2 centre point, 2 end point, 1 concentric, 1 symmetric about line, 1 other
  measures "d172" diameter of A0
extrude "Выдавливание30" cut sketch "Эскиз34" against normal blind 1.5 contours A2
sketch "Эскиз35" plane through (1.5, 0, 0) normal (1, 0, 0) x (0, 0, -1)
  line L0 (37, 163) -> (1, 163) projected
  point P0 (0, 0)
sketch "Эскиз36" plane through (1.5, 0, 0) normal (1, 0, 0) x (0, 0, -1)
  line L0 (-10, 3) -> (-10, 160)
  line L1 (-2, 160) -> (-2, 3)
  arc A0 (-2, 3) -> (1, 0) centre (1, 3) ccw projected
  line L2 (-7, 0) -> (1, 0)
  arc A1 (-2, 3) -> (1, 0) centre (1, 3) ccw
  line L3 (37, 163) -> (1, 163) projected
  line L4 (-7, 163) -> (1, 163)
  arc A2 (1, 163) -> (-2, 160) centre (1, 160) ccw projected
  arc A3 (1, 163) -> (-2, 160) centre (1, 160) ccw
  line L5 (-11, 269.848) -> (-11, 367)
  line L6 (-2, 367) -> (-2, 269.848)
  arc A4 (-2, 269.848) -> (1, 266.848) centre (1, 269.848) ccw projected
  line L7 (1, 266.848) -> (-8, 266.848)
  line L8 (37, 370) -> (1, 370) projected
  line L9 (1.204, 370) -> (-8, 370)
  arc A5 (1, 370) -> (-2, 367) centre (1, 367) ccw
  arc A6 (-2, 269.848) -> (1, 266.848) centre (1, 269.848) ccw
  line L10 (380, 269.848) -> (380, 367)
  line L11 (372, 367) -> (372, 269.848)
  arc A7 (369, 266.848) -> (372, 269.848) centre (369, 269.848) ccw projected
  line L12 (369, 266.848) -> (377, 266.848)
  line L13 (369, 370) -> (333, 370) projected
  line L14 (369, 370) -> (377, 370)
  arc A8 (372, 367) -> (369, 370) centre (369, 367) ccw
  arc A9 (369, 266.848) -> (372, 269.848) centre (369, 269.848) ccw
  line L15 (380, 3) -> (380, 160)
  line L16 (372, 160) -> (372, 3)
  arc A10 (369, 0) -> (372, 3) centre (369, 3) ccw projected
  line L17 (369, 0) -> (377, 0)
  line L18 (369, 163) -> (377, 163)
  arc A11 (372, 160) -> (369, 163) centre (369, 160) ccw projected
  arc A12 (372, 160) -> (369, 163) centre (369, 160) ccw
  arc A13 (369, 0) -> (372, 3) centre (369, 3) ccw
  arc A14 (-8, 370) -> (-11, 367) centre (-8, 367) ccw
  arc A15 (-11, 269.848) -> (-8, 266.848) centre (-8, 269.848) ccw
  arc A16 (-7, 163) -> (-10, 160) centre (-7, 160) ccw
  arc A17 (-10, 3) -> (-7, 0) centre (-7, 3) ccw
  arc A18 (380, 160) -> (377, 163) centre (377, 160) ccw
  arc A19 (377, 0) -> (380, 3) centre (377, 3) ccw
  arc A20 (380, 367) -> (377, 370) centre (377, 367) ccw
  arc A21 (377, 266.848) -> (380, 269.848) centre (377, 269.848) ccw
  point P0 (0, 0)
  point P1 (-10, 163)
  point P2 (-10, 0)
  point P3 (-11, 370)
  point P4 (-11, 266.848)
  point P5 (380, 266.848)
  point P6 (380, 370)
  point P7 (380, 163)
  point P8 (380, 0)
  dimension "d185" = 3
  dimension "d186" = 3
  dimension "d187" = 3
  constraints: 39 point on circle, 32 end point, 24 tangent, 17 point on line, 16 centre point, 7 horizontal, 6 equal radius, 4 parallel, 1 concentric
  measures "d185" radius of A14
  measures "d186" radius of A15
  measures "d187" radius of A21
extrude "Выдавливание31" cut sketch "Эскиз36" against normal blind 1.5
sketch "Эскиз37" plane through (1.5, 0, 0) normal (1, 0, 0) x (0, 0, -1)
  point P0 (0, 0)
sketch "Эскиз38" plane through (1.5, 0, 0) normal (1, 0, 0) x (0, 0, -1)
  circle A0 centre (-1, 228) radius 1.625 projected
  circle A1 centre (-1.0468, 185.0848) radius 1.625 projected
  line L0 (-1.0468, 185.0848) -> (6.9532, 185.0848) construction
  circle A2 centre (-9, 228) radius 1.625
  circle A3 centre (-9.0468, 185.0848) radius 1.625
  circle A4 centre (371.0468, 185.0848) radius 1.625 projected
  circle A5 centre (371, 228) radius 1.625 projected
  circle A6 centre (379, 228) radius 1.625
  circle A7 centre (379.0468, 185.0848) radius 1.625
  circle A8 centre (-1.0468, 185.0848) radius 1.625
  circle A9 centre (-1, 228) radius 1.625
  circle A10 centre (371.0468, 185.0848) radius 1.625
  circle A11 centre (371, 228) radius 1.625
  point P0 (0, 0)
  dimension "d191" = 3.25
  dimension "d192" = 3.25
  dimension "d195" = 3.25
  dimension "d196" = 3.25
  constraints: 8 centre point, 4 coincident, 3 concentric, 2 end point, 1 horizontal
  measures "d191" diameter of A2
  measures "d192" diameter of A3
  measures "d195" diameter of A6
  measures "d196" diameter of A7
extrude "Выдавливание32" cut sketch "Эскиз38" against normal blind 1.5 contours A2 | A3 | A6 | A7
sketch "Эскиз39" plane through (1.5, 0, 0) normal (1, 0, 0) x (0, 0, -1)
  circle A0 centre (-1, 228) radius 1.625 projected
  circle A1 centre (-1, 228) radius 1.625
  circle A2 centre (-1.0468, 185.0848) radius 1.625 projected
  circle A3 centre (-1.0468, 185.0848) radius 1.625
  circle A4 centre (371.0468, 185.0848) radius 1.625 projected
  circle A5 centre (371.0468, 185.0848) radius 1.625
  circle A6 centre (371, 228) radius 1.625
  circle A7 centre (371, 228) radius 1.625 projected
  point P0 (0, 0)
  dimension "d199" = 3.25
  constraints: 4 centre point, 3 coincident, 1 concentric
  measures "d199" diameter of A6
extrude "Выдавливание33" add sketch "Эскиз39" against normal blind 1.5
sketch "Эскиз40" plane through (1.5, 0, 0) normal (1, 0, 0) x (0, 0, -1)
  arc A0 (-10, 3) -> (-7.8605, 0.1261) centre (-7, 3) ccw projected
  arc A1 (-7.8605, 0.1261) -> (-4.2111, 0) centre (-6, 1.1) ccw projected
  circle A2 centre (-13.6, 1.1) radius 1.625
  line L0 (-18, 372) -> (-18, -2) projected
  circle A3 centre (-13.6, 369) radius 1.625
  line L1 (75, 375) -> (-15, 375) projected
  arc A4 (374.2111, 0) -> (377.8605, 0.1261) centre (376, 1.1) ccw projected
  circle A5 centre (383.6, 1.1) radius 1.625
  line L2 (388, -2) -> (388, 372) projected
  arc A6 (377.8605, 369.8739) -> (374.2111, 370) centre (376, 368.9) ccw projected
  circle A7 centre (383.6, 368.9) radius 1.625
  point P0 (0, 0)
  dimension "d203" = 3.25
  dimension "d204" = 4.4
  dimension "d205" = 3.25
  dimension "d206" = 4.4
  dimension "d208" = 6
  dimension "d209" = 3.25
  dimension "d210" = 4.4
  dimension "d212" = 3.25
  dimension "d213" = 4.4
  constraints: 4 centre point, 1 point on circle
  measures "d203" diameter of A2
  measures "d204" distance from line of L0 A2.centre
  measures "d205" diameter of A3
  measures "d206" distance from line of L0 A3.centre
  measures "d208" distance from line of L1 A3.centre
  measures "d209" diameter of A5
  measures "d210" distance from line of L2 A5.centre
  measures "d212" diameter of A7
  measures "d213" distance from line of L2 A7.centre
extrude "Выдавливание34" cut sketch "Эскиз40" against normal blind 1.5